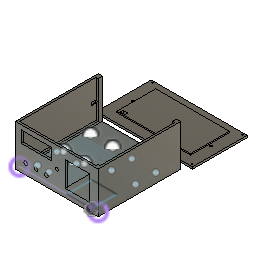
main_unit_box v6 (Autodesk Fusion 360 design; units mm, degrees)
Autodesk Fusion 360 part; units mm, degrees
sketch "Sketch1" plane through (0, 0, 0) normal (0, 0, 1) x (1, 0, 0)
  line L0 (0, 0) -> (-200, 0)
  line L1 (-200, 0) -> (-200, 100)
  line L2 (-200, 100) -> (0, 100)
  line L3 (0, 100) -> (0, 0)
  line L4 (-186.5, 89) -> (-113.5, 89)
  line L5 (-113.5, 89) -> (-113.5, 61)
  line L6 (-113.5, 61) -> (-186.5, 61)
  line L7 (-186.5, 61) -> (-186.5, 89)
  line L8 (-186.5, 89) -> (-113.5, 61) construction
  line L9 (-113.5, 89) -> (-186.5, 61) construction
  line L10 (-80, 20) -> (-20, 20)
  line L11 (-20, 20) -> (-20, 80)
  line L12 (-20, 80) -> (-80, 80)
  line L13 (-80, 80) -> (-80, 20)
  line L14 (-80, 20) -> (-20, 80) construction
  line L15 (-20, 20) -> (-80, 80) construction
  circle A0 centre (-100, 50) radius 4
  circle A1 centre (-175, 25) radius 4.5
  circle A2 centre (-150, 25) radius 4.5
  circle A3 centre (-125, 25) radius 4.5
  point P0 (-150, 75)
  point P1 (-50, 50)
  dimension "d1" = 200
  dimension "d2" = 100
  dimension "d3" = 73
  dimension "d4" = 28
  dimension "d5" = 60
  dimension "d6" = 60
  dimension "d7" = 8
  dimension "d9" = 9
  dimension "d10" = 9
  dimension "d11" = 9
  constraint horizontal L0
  constraint vertical L1
  constraint horizontal L2
  constraint vertical L3
  constraint coincident L0.start L3.end
  constraint horizontal L4
  constraint perpendicular L4 L5
  constraint parallel L4 L6
  constraint parallel L5 L7
  constraint coincident L8 P0
  constraint coincident L9 P0
  constraint horizontal L10
  constraint perpendicular L10 L11
  constraint parallel L10 L12
  constraint parallel L11 L13
  constraint coincident L14 P1
  constraint coincident L15 P1
  measures "d1" distance of L0.start L0.end
  measures "d2" distance of L0.start L2.end
  measures "d3" distance of L5.end L6.end
  measures "d4" distance of L4.end L5.end
  measures "d5" distance of L11.end L12.end
  measures "d6" distance of L10.end L11.end
  measures "d7" diameter of A0
  measures "d9" diameter of A1
  measures "d10" diameter of A2
  measures "d11" diameter of A3
extrude "Extrude1" add sketch "Sketch1" along normal blind 5 makes body 1
move_body "Move1" bodies 1 to x (1, 0, 0) y (0, 0, 1) z (0, -1, 0) at (0, 46.5537, -36.5537)
move_body "Move2" bodies 1 to x (1, 0, 0) y (0, 1, 0) z (0, 0, 1) at (0, 0, 35)
sketch "Sketch2" plane through (0, 46.5537, 0) normal (0, 1, 0) x (-1, 0, 0)
  line L0 (80, 78.4463) -> (80, 18.4463)
  line L1 (80, 18.4463) -> (20, 18.4463)
  line L2 (20, 18.4463) -> (20, 78.4463)
  line L3 (20, 78.4463) -> (80, 78.4463)
  circle A0 centre (100, 48.4463) radius 4
  circle A1 centre (125, 23.4463) radius 4.5
  circle A2 centre (175, 23.4463) radius 4.5
  line L4 (186.5, 59.4463) -> (113.5, 59.4463)
  line L5 (113.5, 59.4463) -> (113.5, 87.4463)
  line L6 (113.5, 87.4463) -> (186.5, 87.4463)
  line L7 (186.5, 87.4463) -> (186.5, 59.4463)
  circle A3 centre (150, 23.4463) radius 4.5
  line L8 (200, 98.4463) -> (0, 98.4463)
  line L9 (0, 98.4463) -> (0, -1.5537)
  line L10 (0, -1.5537) -> (200, -1.5537)
  line L11 (200, -1.5537) -> (200, 98.4463)
  line L12 (0, 98.4463) -> (5, 98.4463)
  line L13 (5, 98.4463) -> (5, -1.5537)
  line L14 (5, -1.5537) -> (0, -1.5537)
  line L15 (0, -1.5537) -> (0, 98.4463)
  line L16 (5, -1.5537) -> (200, -1.5537)
  line L17 (200, -1.5537) -> (200, 3.4463)
  line L18 (200, 3.4463) -> (5, 3.4463)
  line L19 (5, 3.4463) -> (5, -1.5537)
  line L20 (200, 3.4463) -> (195, 3.4463)
  line L21 (195, 3.4463) -> (195, 98.4463)
  line L22 (195, 98.4463) -> (200, 98.4463)
  line L23 (200, 98.4463) -> (200, 3.4463)
  dimension "d14" = 5
  dimension "d15" = 5
  dimension "d16" = 5
  constraint horizontal L12
  constraint vertical L13
  constraint horizontal L14
  constraint vertical L15
  constraint coincident L8.end L9.start
  constraint horizontal L16
  constraint vertical L17
  constraint horizontal L18
  constraint vertical L19
  constraint horizontal L20
  constraint vertical L21
  constraint horizontal L22
  constraint vertical L23
  measures "d14" distance of L8.end L12.end
  measures "d15" distance of L13.end L18.end
  measures "d16" distance of L17.end L20.end
extrude "Extrude2" add sketch "Sketch2" along normal blind 140 contours L8 L11 L18 L20 L21 L22 L23 | L10 L11 L13 L16 L17 L18 L19 L20 | L8 L9 L10 L12 L13 L14 L15 L19 bodies 1
sketch "Sketch3" plane through (0, 0, 3.4463) normal (0, 0, 1) x (-1, 0, 0)
  line L0 (195, -46.5537) -> (5, -46.5537)
  line L1 (5, -46.5537) -> (5, -186.5537)
  line L2 (5, -186.5537) -> (195, -186.5537)
  line L3 (195, -186.5537) -> (195, -46.5537)
  circle A0 centre (76, -199) radius 3
  circle A1 centre (76, -150) radius 3
  circle A2 centre (18, -199) radius 3
  circle A3 centre (18, -150) radius 3
  line L4 (175, -131.42) -> (172.46, -131.42)
  line L5 (121.66, -131.42) -> (124.2, -131.42)
  line L6 (175, -197.46) -> (175, -200)
  line L7 (121.66, -197.46) -> (121.66, -200)
  circle A4 centre (132.84, -121.66) radius 3
  circle A5 centre (181.1, -122.93) radius 3
  circle A6 centre (148.08, -70.86) radius 3
  circle A7 centre (176.02, -70.86) radius 3
  dimension "d20" = 6
  dimension "d21" = 49
  dimension "d22" = 6
  dimension "d23" = 58
  dimension "d24" = 6
  dimension "d25" = 49
  dimension "d26" = 6
  dimension "d32" = 53.34
  dimension "d33" = 68.58
  dimension "d34" = 2.54
  dimension "d36" = 2.54
  dimension "d39" = 2.54
  dimension "d41" = 2.54
  dimension "d42" = 6
  dimension "d43" = 6
  dimension "d44" = 6
  dimension "d45" = 6
  constraint horizontal L4
  constraint horizontal L5
  constraint vertical L6
  constraint vertical L7
  measures "d20" diameter of A0
  measures "d21" distance of A0.centre A1.centre
  measures "d22" diameter of A1
  measures "d23" distance of A0.centre A2.centre
  measures "d24" diameter of A2
  measures "d25" distance of A2.centre A3.centre
  measures "d26" diameter of A3
  measures "d32" distance of L6.end L7.end
  measures "d33" distance of L6.end L4.start
  measures "d34" distance of L4.start L4.end
  measures "d36" distance of L5.start L5.end
  measures "d39" distance of L6.end L6.start
  measures "d41" distance of L7.end L7.start
  measures "d42" diameter of A4
  measures "d43" diameter of A5
  measures "d44" diameter of A6
  measures "d45" diameter of A7
sketch "Sketch4" plane through (0, 0, 3.4463) normal (0, 0, 1) x (-1, 0, 0)
  line L0 (19.9409, -46.5537) -> (79.9409, -46.5537)
  line L1 (79.9409, -46.5537) -> (79.9409, -106.5537)
  line L2 (79.9409, -106.5537) -> (19.9409, -106.5537)
  line L3 (19.9409, -106.5537) -> (19.9409, -46.5537)
  line L4 (5, -46.5537) -> (195, -46.5537)
  dimension "d46" = 60
  dimension "d47" = 60
  constraint horizontal L0
  constraint vertical L1
  constraint horizontal L2
  constraint vertical L3
  constraint coincident L0.start L4
  measures "d46" distance of L0.start L0.end
  measures "d47" distance of L0.start L2.end
extrude "Extrude3" add sketch "Sketch4" along normal blind 10 bodies 1
extrude "Extrude4" add 1 faces at (-68.3333, 186.5537, 0.113) along direction (0, 1, 0) blind 50 on bodies 1 bodies 1
sketch "Sketch5" plane through (0, 0, 3.4463) normal (0, 0, 1) x (-1, 0, 0)
  line L0 (79.9409, -46.5537) -> (79.9409, -106.5537)
  line L1 (79.9409, -106.5537) -> (19.9409, -106.5537)
  line L2 (19.9409, -106.5537) -> (19.9409, -46.5537)
  line L3 (19.9409, -46.5537) -> (5, -46.5537)
  line L4 (5, -46.5537) -> (5, -236.5537)
  line L5 (5, -236.5537) -> (195, -236.5537)
  line L6 (195, -236.5537) -> (195, -46.5537)
  line L7 (195, -46.5537) -> (79.9409, -46.5537)
extrude "Extrude5" add sketch "Sketch3" along normal blind 5 contours A0 | A1 | A2 | A3 bodies 1
sketch "Sketch6" plane through (0, 46.5537, 0) normal (0, 1, 0) x (-1, 0, 0)
  line L0 (79.9409, 13.4463) -> (79.9409, 3.4463)
  line L1 (79.9409, 3.4463) -> (195, 3.4463)
  line L2 (195, 3.4463) -> (195, 98.4463)
  line L3 (195, 98.4463) -> (5, 98.4463)
  line L4 (5, 98.4463) -> (5, 3.4463)
  line L5 (5, 3.4463) -> (19.9409, 3.4463)
  line L6 (19.9409, 3.4463) -> (19.9409, 13.4463)
  line L7 (19.9409, 13.4463) -> (79.9409, 13.4463)
  circle A0 centre (150, 23.4463) radius 4.5
  line L8 (186.5, 59.4463) -> (113.5, 59.4463)
  line L9 (113.5, 59.4463) -> (113.5, 87.4463)
  line L10 (113.5, 87.4463) -> (186.5, 87.4463)
  line L11 (186.5, 87.4463) -> (186.5, 59.4463)
  circle A1 centre (175, 23.4463) radius 4.5
  circle A2 centre (125, 23.4463) radius 4.5
  circle A3 centre (100, 48.4463) radius 4
  line L12 (80, 78.4463) -> (80, 18.4463)
  line L13 (80, 18.4463) -> (20, 18.4463)
  line L14 (20, 18.4463) -> (20, 78.4463)
  line L15 (20, 78.4463) -> (80, 78.4463)
  line L16 (5, 3.4463) -> (10, 3.4463)
  line L17 (10, 3.4463) -> (10, 8.4463)
  line L18 (10, 8.4463) -> (5, 8.4463)
  line L19 (5, 8.4463) -> (5, 3.4463)
  line L20 (195, 3.4463) -> (190, 3.4463)
  line L21 (190, 3.4463) -> (190, 8.4463)
  line L22 (190, 8.4463) -> (195, 8.4463)
  line L23 (195, 8.4463) -> (195, 3.4463)
  dimension "d56" = 5
  dimension "d57" = 5
  dimension "d58" = 5
  dimension "d59" = 5
  constraint horizontal L16
  constraint vertical L17
  constraint horizontal L18
  constraint vertical L19
  constraint coincident L4.end L5.start
  constraint horizontal L20
  constraint vertical L21
  constraint horizontal L22
  constraint vertical L23
  constraint coincident L1.end L2.start
  measures "d56" distance of L4.end L16.end
  measures "d57" distance of L4.end L18.end
  measures "d58" distance of L1.end L20.end
  measures "d59" distance of L1.end L22.end
extrude "Extrude7" add sketch "Sketch6" along normal blind 190 contours L1 L2 L20 L21 L22 L23 | L4 L5 L16 L17 L18 L19 bodies 1
sketch "Sketch7" plane through (0, 0, 8.4463) normal (0, 0, 1) x (-1, 0, 0)
  line L0 (10, -46.5537) -> (5, -46.5537)
  line L1 (5, -46.5537) -> (5, -236.5537)
  line L2 (5, -236.5537) -> (10, -236.5537)
  line L3 (10, -236.5537) -> (10, -46.5537)
  line L4 (10, -236.5537) -> (5, -236.5537)
  line L5 (5, -236.5537) -> (5, -231.5537)
  line L6 (5, -231.5537) -> (10, -231.5537)
  line L7 (10, -231.5537) -> (10, -236.5537)
  dimension "d62" = 5
  dimension "d63" = 5
  constraint horizontal L4
  constraint vertical L5
  constraint horizontal L6
  constraint vertical L7
  constraint coincident L2.end L3.start
  measures "d62" distance of L2.end L1.end
  measures "d63" distance of L2.end L6.end
sketch "Sketch8" plane through (0, 0, 8.4463) normal (0, 0, 1) x (-1, 0, 0)
  line L0 (195, -46.5537) -> (190, -46.5537)
  line L1 (190, -46.5537) -> (190, -236.5537)
  line L2 (190, -236.5537) -> (195, -236.5537)
  line L3 (195, -236.5537) -> (195, -46.5537)
  line L4 (195, -236.5537) -> (190, -236.5537)
  line L5 (190, -236.5537) -> (190, -231.5537)
  line L6 (190, -231.5537) -> (195, -231.5537)
  line L7 (195, -231.5537) -> (195, -236.5537)
  dimension "d64" = 5
  dimension "d65" = 5
  constraint horizontal L4
  constraint vertical L5
  constraint horizontal L6
  constraint vertical L7
  constraint coincident L2.end L3.start
  measures "d64" distance of L2.end L1.end
  measures "d65" distance of L2.end L6.end
extrude "Extrude8" add sketch "Sketch7" sketch "Sketch8" along normal blind 90 contours L1 L2 L3 L4 L5 L6 L7 of sketch 2 contours L1 L2 L3 L4 L5 L6 L7 bodies 1
sketch "Sketch9" plane through (0, 0, 0) normal (0, 0, 1) x (1, 0, 0)
  line L0 (-200, 270) -> (0, 270)
  line L1 (0, 270) -> (0, 370)
  line L2 (0, 370) -> (-200, 370)
  line L3 (-200, 370) -> (-200, 270)
  dimension "d68" = 200
  dimension "d69" = 100
  constraint horizontal L0
  constraint vertical L1
  constraint horizontal L2
  constraint vertical L3
  measures "d68" distance of L0.start L0.end
  measures "d69" distance of L0.start L2.end
extrude "Extrude9" add sketch "Sketch9" along normal blind 5 separate body makes body 2
sketch "Sketch10" plane through (0, 0, 5) normal (0, 0, 1) x (-1, 0, 0)
  line L0 (200, -370) -> (200, -270)
  line L1 (200, -270) -> (0, -270)
  line L2 (0, -270) -> (0, -370)
  line L3 (0, -370) -> (200, -370)
  line L4 (189, -276) -> (11, -276)
  line L5 (11, -276) -> (11, -364)
  line L6 (11, -364) -> (189, -364)
  line L7 (189, -364) -> (189, -276)
  line L8 (11, -364) -> (189, -364)
  line L9 (189, -364) -> (189, -370)
  line L10 (189, -370) -> (11, -370)
  line L11 (11, -370) -> (11, -364)
  point P0 (100, -320)
  dimension "d72" = 178
  dimension "d73" = 88
  constraint horizontal L4
  constraint perpendicular L4 L5
  constraint parallel L4 L6
  constraint parallel L5 L7
  constraint horizontal L8
  constraint vertical L9
  constraint horizontal L10
  constraint vertical L11
  constraint coincident L3 L9.end
  measures "d72" distance of L5.end L6.end
  measures "d73" distance of L4.end L5.end
extrude "Extrude10" add sketch "Sketch10" along normal blind 3 contours L3 L6 L8 L9 L10 L11 | L4 L5 L6 L7 L8 bodies 2
sketch "Sketch11" plane through (0, 0, 5) normal (0, 0, 1) x (-1, 0, 0)
  line L0 (11, -370) -> (11, -276)
  line L1 (11, -276) -> (189, -276)
  line L2 (189, -276) -> (189, -364)
  line L3 (189, -364) -> (189, -370)
  line L4 (189, -370) -> (200, -370)
  line L5 (200, -370) -> (200, -270)
  line L6 (200, -270) -> (0, -270)
  line L7 (0, -270) -> (0, -370)
  line L8 (0, -370) -> (11, -370)
  circle A0 centre (194.5, -320) radius 2.5
  circle A1 centre (5.5, -320) radius 2.5
  dimension "d77" = 5
  dimension "d78" = 5
  measures "d77" diameter of A0
  measures "d78" diameter of A1
extrude "Extrude11" cut sketch "Sketch11" against normal blind 5 contours A0 | A1 bodies 2
sketch "Sketch12" plane through (0, 236.5537, 0) normal (0, 1, 0) x (-1, 0, 0)
  line L0 (190, 3.4463) -> (10, 3.4463)
  line L1 (10, 3.4463) -> (10, 98.4463)
  line L2 (10, 98.4463) -> (0, 98.4463)
  line L3 (0, 98.4463) -> (0, -1.5537)
  line L4 (0, -1.5537) -> (200, -1.5537)
  line L5 (200, -1.5537) -> (200, 98.4463)
  line L6 (200, 98.4463) -> (190, 98.4463)
  line L7 (190, 98.4463) -> (190, 3.4463)
sketch "Sketch13" plane through (0, 236.5537, 0) normal (0, 1, 0) x (-1, 0, 0)
  line L0 (0, -1.5537) -> (200, -1.5537)
  circle A0 centre (5, 48.4463) radius 2.5
  circle A1 centre (195, 48.1649) radius 2.5
  point P0 (10, 98.4463)
  point P1 (0, -1.5537)
  point P2 (0, 98.4463)
  point P3 (200, 98.4463)
  dimension "d81" = 5
  dimension "d82" = 5
  measures "d81" diameter of A0
  measures "d82" diameter of A1
extrude "Extrude12" cut sketch "Sketch13" against normal blind 5 bodies 1
sketch "Sketch14" plane through (0, 0, 8.4463) normal (0, 0, 1) x (-1, 0, 0)
  line L0 (190, -231.5537) -> (195, -231.5537)
  line L1 (195, -231.5537) -> (195, -46.5537)
  line L2 (195, -46.5537) -> (190, -46.5537)
  line L3 (190, -46.5537) -> (190, -231.5537)
  line L4 (195, -46.5537) -> (190, -46.5537)
  line L5 (190, -46.5537) -> (190, -51.5537)
  line L6 (190, -51.5537) -> (195, -51.5537)
  line L7 (195, -51.5537) -> (195, -46.5537)
  dimension "d85" = 5
  constraint horizontal L4
  constraint vertical L5
  constraint horizontal L6
  constraint vertical L7
  constraint coincident L1.end L2.start
  measures "d85" distance of L1.end L6.end
sketch "Sketch15" plane through (0, 0, 8.4463) normal (0, 0, 1) x (-1, 0, 0)
  line L0 (5, -231.5537) -> (10, -231.5537)
  line L1 (10, -231.5537) -> (10, -46.5537)
  line L2 (10, -46.5537) -> (5, -46.5537)
  line L3 (5, -46.5537) -> (5, -231.5537)
  line L4 (5, -46.5537) -> (10, -46.5537)
  line L5 (10, -46.5537) -> (10, -51.5537)
  line L6 (10, -51.5537) -> (5, -51.5537)
  line L7 (5, -51.5537) -> (5, -46.5537)
  dimension "d86" = 5
  constraint horizontal L4
  constraint vertical L5
  constraint horizontal L6
  constraint vertical L7
  constraint coincident L2.end L3.start
  measures "d86" distance of L2.end L6.end
extrude "Extrude13" add sketch "Sketch15" along normal blind 90 contours L1 L2 L3 L4 L5 L6 L7 bodies 1
extrude "Extrude14" add sketch "Sketch14" along normal blind 40 contours L1 L2 L3 L4 L5 L6 L7 bodies 1
sketch "Sketch16" plane through (-195, 0, 0) normal (1, 0, 0) x (0, 1, 0)
  line L0 (51.5537, 48.4463) -> (51.5537, 8.4463)
  line L1 (51.5537, 8.4463) -> (231.5537, 8.4463)
  line L2 (231.5537, 8.4463) -> (231.5537, 45.6649)
  line L3 (231.5537, 45.6649) -> (231.5537, 50.6649)
  line L4 (231.5537, 50.6649) -> (231.5537, 98.4463)
  line L5 (231.5537, 98.4463) -> (46.5537, 98.4463)
  line L6 (46.5537, 98.4463) -> (46.5537, 48.4463)
  line L7 (46.5537, 48.4463) -> (51.5537, 48.4463)
  line L8 (231.5537, 51.3437) -> (221.5537, 51.3437)
  line L9 (221.5537, 51.3437) -> (221.5537, 44.3437)
  line L10 (221.5537, 44.3437) -> (231.5537, 44.3437)
  line L11 (231.5537, 44.3437) -> (231.5537, 51.3437)
  dimension "d91" = 10
  dimension "d92" = 7
  constraint horizontal L8
  constraint vertical L9
  constraint horizontal L10
  constraint vertical L11
  constraint coincident L4 L8.start
  measures "d91" distance of L8.start L8.end
  measures "d92" distance of L8.start L10.end
extrude "Extrude15" cut sketch "Sketch16" against normal blind 2 contours L2 L3 L4 L8 L9 L10 L11 bodies 1
sketch "Sketch17" plane through (-5, 0, 0) normal (-1, 0, 0) x (0, -1, 0)
  line L0 (-51.5537, 8.4463) -> (-51.5537, 98.4463)
  line L1 (-51.5537, 98.4463) -> (-231.5537, 98.4463)
  line L2 (-231.5537, 98.4463) -> (-231.5537, 50.9463)
  line L3 (-231.5537, 50.9463) -> (-231.5537, 45.9463)
  line L4 (-231.5537, 45.9463) -> (-231.5537, 8.4463)
  line L5 (-231.5537, 8.4463) -> (-51.5537, 8.4463)
  line L6 (-231.5537, 51.5702) -> (-221.5537, 51.5702)
  line L7 (-221.5537, 51.5702) -> (-221.5537, 45.5702)
  line L8 (-221.5537, 45.5702) -> (-231.5537, 45.5702)
  line L9 (-231.5537, 45.5702) -> (-231.5537, 51.5702)
  dimension "d95" = 10
  dimension "d96" = 6
  constraint horizontal L6
  constraint vertical L7
  constraint horizontal L8
  constraint vertical L9
  constraint coincident L2 L6.start
  measures "d95" distance of L6.start L6.end
  measures "d96" distance of L6.start L8.end
extrude "Extrude16" cut sketch "Sketch17" against normal blind 2 contours L2 L3 L4 L6 L7 L8 L9 bodies 1
sketch "Sketch18" plane through (0, 0, 8.4463) normal (0, 0, 1) x (-1, 0, 0)
  circle A0 centre (18, -199) radius 3
  circle A1 centre (18, -199) radius 1.5
  circle A2 centre (74, -137) radius 1.5
  circle A3 centre (74, -195) radius 1.5
  circle A4 centre (25, -195) radius 1.5
  dimension "d101" = 3
  dimension "d102" = 3
  dimension "d103" = 3
  dimension "d104" = 3
  constraint concentric A0 A1
  measures "d101" diameter of A1
  measures "d102" diameter of A2
  measures "d103" diameter of A3
  measures "d104" diameter of A4
sketch "Sketch19" plane through (0, 0, 8.4463) normal (0, 0, 1) x (-1, 0, 0)
  circle A0 centre (76, -199) radius 3
  circle A1 centre (25, -137) radius 1.25
  circle A2 centre (74, -137) radius 1.25
  circle A3 centre (74, -195) radius 1.25
  circle A4 centre (76, -199) radius 1.25
  dimension "d105" = 2.5
  dimension "d106" = 2.5
  dimension "d107" = 2.5
  dimension "d108" = 2.5
  constraint concentric A0 A4
  measures "d105" diameter of A1
  measures "d106" diameter of A2
  measures "d107" diameter of A3
  measures "d108" diameter of A4
extrude "Extrude17" add sketch "Sketch3" along normal blind 5 contours A4 | A5 | A6 | A7 bodies 1
sketch "Sketch20" plane through (0, 0, 8.4463) normal (0, 0, 1) x (-1, 0, 0)
  circle A0 centre (132.84, -121.66) radius 3
  circle A1 centre (132.84, -121.66) radius 1.5
  circle A2 centre (172.5, -145.5) radius 1.5
  circle A3 centre (167.5, -197.5) radius 1.5
  circle A4 centre (139.5, -197.5) radius 1.5
  dimension "d111" = 3
  dimension "d112" = 3
  dimension "d113" = 3
  dimension "d114" = 3
  constraint concentric A0 A1
  measures "d111" diameter of A1
  measures "d112" diameter of A2
  measures "d113" diameter of A3
  measures "d114" diameter of A4
sketch "Sketch21" plane through (0, 370, 0) normal (0, 1, 0) x (-1, 0, 0)
  line L0 (0, 0) -> (200, 0)
  line L1 (200, 0) -> (200, 5)
  line L2 (200, 5) -> (189, 5)
  line L3 (189, 5) -> (189, 8)
  line L4 (189, 8) -> (11, 8)
  line L5 (11, 8) -> (11, 5)
  line L6 (11, 5) -> (0, 5)
  line L7 (0, 5) -> (0, 0)
  line L8 (11, 5) -> (189, 5)
  constraint coincident L5.end L6.start
  constraint coincident L2.end L3.start
extrude "Extrude19" add sketch "Sketch21" along normal blind 16 contours L0 L1 L2 L6 L7 L8 bodies 2
extrude "Extrude20" add 1 faces at (0, 347.3333, 3.3333) along direction (1, 0, 0) blind 16 on bodies 2 bodies 2
extrude "Extrude21" add 1 faces at (-200, 347.3333, 1.6667) along direction (-1, 0, 0) blind 16 on bodies 2 bodies 2
extrude "Extrude22" add 1 faces at (-138.6667, 270, 3.3333) along direction (0, -1, 0) blind 16 on bodies 2 bodies 2
extrude "Extrude23" add 1 faces at (-195, 236.5537, 82.5192) along direction (0, 1, 0) blind 5 on bodies 1 bodies 1
sketch "Sketch22" plane through (0, 0, 8) normal (0, 0, 1) x (-1, 0, 0)
  line L0 (189, -364) -> (189, -276)
  line L1 (189, -276) -> (11, -276)
  line L2 (11, -276) -> (11, -370)
  line L3 (11, -370) -> (189, -370)
  line L4 (189, -370) -> (189, -364)
  line L5 (172.125, -285.375) -> (183.625, -285.375)
  line L6 (183.625, -285.375) -> (183.625, -278.375)
  line L7 (183.625, -278.375) -> (172.125, -278.375)
  line L8 (172.125, -278.375) -> (172.125, -285.375)
  line L9 (172.125, -285.375) -> (183.625, -278.375) construction
  line L10 (183.625, -285.375) -> (172.125, -278.375) construction
  point P0 (177.875, -281.875)
  dimension "d127" = 11.5
  dimension "d128" = 7
  constraint horizontal L5
  constraint perpendicular L5 L6
  constraint parallel L5 L7
  constraint parallel L6 L8
  constraint coincident L9 P0
  constraint coincident L10 P0
  measures "d127" distance of L6.end L7.end
  measures "d128" distance of L5.end L6.end
extrude "Extrude24" cut sketch "Sketch22" against normal blind 10 contours L5 L6 L7 L8 bodies 2
extrude "Extrude25" add 1 faces at (-39.9409, 66.5537, 13.4463) along direction (0, 0, 1) blind 4 on bodies 1 bodies 1
extrude "Extrude26" add 1 faces at (-39.9409, 66.5537, 17.4463) along direction (0, 0, 1) blind 1 on bodies 1 bodies 1
sketch "Sketch23" plane through (0, 0, 8.4463) normal (0, 0, 1) x (-1, 0, 0)
  circle A0 centre (18, -150) radius 3
sketch "Sketch24" plane through (0, 0, 8.4463) normal (0, 0, 1) x (-1, 0, 0)
  circle A0 centre (76, -150) radius 3
  circle A1 centre (76, -150) radius 1.25
  circle A2 centre (18, -150) radius 1.25
  circle A3 centre (18, -199) radius 1.25
  circle A4 centre (76, -199) radius 1.25
  circle A5 centre (132.8427, -121.6631) radius 1.5
  circle A6 centre (181.1073, -122.9314) radius 1.5
  circle A7 centre (176.0205, -70.8633) radius 1.5
  circle A8 centre (148.0698, -70.8619) radius 1.5
  point P0 (18, -150)
  dimension "d135" = 2.5
  dimension "d136" = 2.5
  dimension "d137" = 2.5
  dimension "d138" = 2.5
  dimension "d140" = 3
  dimension "d141" = 3
  dimension "d142" = 3
  dimension "d143" = 3
  constraint concentric A0 A1
  constraint coincident P0 A2.centre
  measures "d135" diameter of A1
  measures "d136" diameter of A2
  measures "d137" diameter of A3
  measures "d138" diameter of A4
  measures "d140" diameter of A5
  measures "d141" diameter of A6
  measures "d142" diameter of A7
  measures "d143" diameter of A8
extrude "Extrude27" cut sketch "Sketch24" against normal blind 7 contours A1 | A2 | A3 | A4 | A5 | A6 | A7 | A8 bodies 1
sketch "Sketch25" plane through (0, 0, 5) normal (0, 0, 1) x (-1, 0, 0)
  line L0 (-16, -254) -> (-16, -386)
  line L1 (-16, -386) -> (216, -386)
  line L2 (216, -386) -> (216, -254)
  line L3 (216, -254) -> (-16, -254)
  circle A0 centre (194.5, -320) radius 2.5
  circle A1 centre (5.5, -320) radius 2.5
  line L4 (189, -370) -> (11, -370)
  line L5 (11, -370) -> (11, -276)
  line L6 (11, -276) -> (189, -276)
  line L7 (189, -276) -> (189, -364)
  line L8 (189, -364) -> (189, -370)
  circle A2 centre (-9.25, -259.5) radius 1.5
  circle A3 centre (209.25, -259.5) radius 1.5
  circle A4 centre (209.25, -382) radius 1.5
  circle A5 centre (-9.25, -382) radius 1.5
  dimension "d146" = 3
  dimension "d147" = 3
  dimension "d148" = 3
  dimension "d149" = 3
  measures "d146" diameter of A2
  measures "d147" diameter of A3
  measures "d148" diameter of A4
  measures "d149" diameter of A5
extrude "Extrude28" cut sketch "Sketch25" against normal blind 10 contours A2 | A3 | A4 | A5 bodies 2
equation "button_diameter = 9 mm"
equation "d9 = button_diameter"
equation "d10 = button_diameter"
equation "d11 = button_diameter"
equation "rpi_screw_hole = 6 mm"
equation "d20 = rpi_screw_hole"
equation "d22 = rpi_screw_hole"
equation "d24 = rpi_screw_hole"
equation "d26 = rpi_screw_hole"
equation "arduino_scre_hole = 6 mm"
equation "d42 = arduino_scre_hole"
equation "d43 = arduino_scre_hole"
equation "d44 = arduino_scre_hole"
equation "d45 = arduino_scre_hole"
equation "back_cover_screw_hole = 5 mm"
equation "d77 = back_cover_screw_hole"
equation "d78 = back_cover_screw_hole"
equation "d81 = back_cover_screw_hole"
equation "d82 = back_cover_screw_hole"
equation "rpi_screw_inner = 2.5 mm"
equation "arduino_screw_inner = 3 mm"
equation "d101 = arduino_screw_inner"
equation "d102 = arduino_screw_inner"
equation "d103 = arduino_screw_inner"
equation "d104 = arduino_screw_inner"
equation "d105 = rpi_screw_inner"
equation "d106 = rpi_screw_inner"
equation "d107 = rpi_screw_inner"
equation "d108 = rpi_screw_inner"
equation "d111 = arduino_screw_inner"
equation "d112 = arduino_screw_inner"
equation "d113 = arduino_screw_inner"
equation "d114 = arduino_screw_inner"
equation "d135 = rpi_screw_inner"
equation "d136 = rpi_screw_inner"
equation "d137 = rpi_screw_inner"
equation "d138 = rpi_screw_inner"
equation "d140 = arduino_screw_inner"
equation "d141 = arduino_screw_inner"
equation "d142 = arduino_screw_inner"
equation "d143 = arduino_screw_inner"
